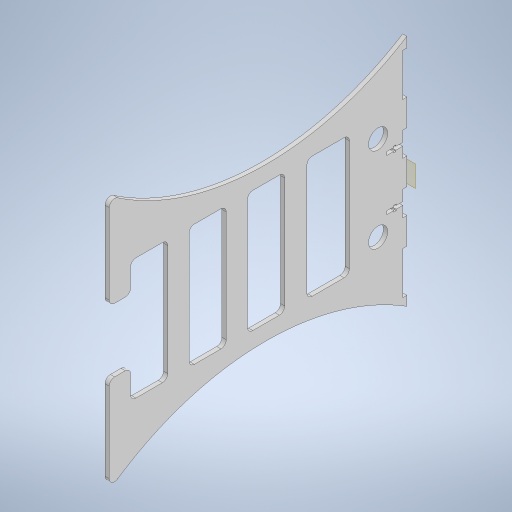
# Autodesk Inventor part: грань тела
Saved by Autodesk Inventor 2023.1 (Build 271208000, 208)
## iProperties
Created: 2024-11-21
Part Number: грань тела
Material: Типовые
Document SubType Name: Modeling
Designer: DELL
Density: 1 g/cm^3
Appearance: По умолчанию
Author: DELL
Autodesk Inventor part; units mm, degrees
ref_plane "YZ Plane" through (0, 0, 0) normal (1, 0, 0) x (0, 1, 0)
ref_plane "XZ Plane" through (0, 0, 0) normal (0, 1, 0) x (-1, 0, 0)
ref_plane "РабПлоскость1" through (0, 0, -4) normal (0, 0, 1) x (1, 0, 0)
sketch "Эскиз10" plane through (0, 0, 0) normal (1, 0, 0) x (0, 1, 0)
  line L0 (-120, -4) -> (120, -4) construction
  line L1 (120, -4) -> (120, 276) construction
  line L2 (110.389, 276) -> (-110.389, 276)
  line L3 (-120, 276) -> (-120, -4) construction
  line L4 (-110, -4) -> (110, -4)
  arc A0 (-110, -4) -> (-114.5368, 268.208) centre (-321.9309, 128.6096) ccw
  arc A1 (114.5368, 268.208) -> (110, -4) centre (321.9309, 128.6096) ccw
  arc A2 (114.5368, 268.208) -> (110.389, 276) centre (110.389, 271) ccw
  arc A3 (-110.389, 276) -> (-114.5368, 268.208) centre (-110.389, 271) ccw
  point P0 (0, 0)
  point P1 (0, -4)
  dimension "d50" = 240
  dimension "d51" = 280
  dimension "d52" = 220
  dimension "d53" = 250
  dimension "d54" = 250
  dimension "d55" = 5
  constraints: 10 end point, 10 point on circle, 4 centre point, 4 tangent, 2 horizontal, 2 midpoint, 2 parallel, 2 point on line, 1 equal radius, 1 perpendicular
  measures "d50" distance of L3.start L1.end
  measures "d51" distance of L1.end L0.end
  measures "d52" distance of L4.start L4.end
  measures "d53" radius of A0
  measures "d54" radius of A1
  measures "d55" radius of A2
extrude "Выдавливание6" add sketch "Эскиз10" along normal mid plane 4
sketch "Эскиз12" plane through (2, 0, 0) normal (1, 0, 0) x (0, 0, -1)
  line L0 (4.1067, -100.9593) -> (0, -100.9593)
  line L1 (0, -100.9593) -> (0, -60.9593)
  line L2 (0, -60.9593) -> (4, -60.9593)
  line L3 (4, 110) -> (4, -110) projected
  line L4 (4, -110) -> (4, 110) projected
  line L5 (4, -35.9593) -> (0, -35.9593)
  line L6 (0, -35.9593) -> (0, -12.5)
  line L7 (0, -12.5) -> (4, -12.5)
  line L8 (4, 12.5) -> (0, 12.5)
  line L9 (0, 12.5) -> (0, 35.5004)
  line L10 (0, 35.5004) -> (4, 35.5004)
  line L11 (4, 60.5004) -> (0, 60.5004)
  line L12 (0, 60.5004) -> (0, 100.5004)
  line L13 (0, 100.5004) -> (4, 100.5004)
  point P0 (0, 0)
  point P1 (4, 12.5)
  point P2 (4, 35.5004)
  point P3 (4, -35.9593)
  point P4 (4, -12.5)
  point P5 (4, -100.9593)
  constraints: 24 end point, 10 perpendicular, 7 point on line, 2 horizontal, 8 other
extrude "Выдавливание7" cut sketch "Эскиз12" against normal blind 4
sketch "Эскиз13" plane through (2, 0, 0) normal (1, 0, 0) x (0, 0, -1)
  line L0 (-15, -22.6546) -> (-15, -25.8046)
  line L1 (0, -25.7683) -> (0, -22.691)
  line L2 (0, -35.9593) -> (0, -12.5) projected
  line L3 (-6.1608, -27.016) -> (-8.4608, -27.016)
  line L4 (-8.4608, -21.516) -> (-6.1608, -21.516)
  line L5 (-15, -24.2296) -> (0, -24.2296) construction
  line L6 (0, -12.5) -> (0, -35.9593) projected
  line L7 (-8.4608, -27.016) -> (-8.4608, -25.8046)
  line L8 (-8.4608, -22.6546) -> (-8.4608, -21.516)
  line L9 (-15, -25.8046) -> (-8.4608, -25.8046)
  line L10 (-6.1608, -25.7683) -> (0, -25.7683)
  line L11 (-6.1608, -21.516) -> (-6.1608, -22.691)
  line L12 (-6.1608, -25.7683) -> (-6.1608, -27.016)
  line L13 (0, -22.691) -> (-6.1608, -22.691)
  line L14 (-8.4608, -22.6546) -> (-15, -22.6546)
  line L15 (0, 12.5) -> (0, 35.5004) projected
  line L16 (0, 18.7449) -> (0, 30.6124)
  line L17 (0, 22.4252) -> (0, 25.5752)
  line L18 (-15, 25.5752) -> (-15, 22.4252)
  line L19 (-8.65, 21.2502) -> (-6.35, 21.2502)
  line L20 (-6.35, 26.7502) -> (-8.65, 26.7502)
  line L21 (-15, 24.0002) -> (0, 24.0002) construction
  line L22 (-8.65, 26.7502) -> (-8.65, 25.5752)
  line L23 (-8.65, 22.4252) -> (-8.65, 21.2502)
  line L24 (-15, 22.4252) -> (-8.65, 22.4252)
  line L25 (-6.35, 22.4252) -> (0, 22.4252)
  line L26 (-6.35, 21.2502) -> (-6.35, 22.4252)
  line L27 (-6.35, 25.5752) -> (-6.35, 26.7502)
  line L28 (0, 25.5752) -> (-6.35, 25.5752)
  line L29 (-8.65, 25.5752) -> (-15, 25.5752)
  circle A0 centre (-23.1563, -40) radius 9
  line L30 (4, -35.9593) -> (4, -60.9593) projected
  line L31 (4, 35.5004) -> (4, 60.5004) projected
  line L32 (0, 0) -> (-64.5188, 0) construction
  circle A1 centre (-23.1563, 40) radius 9
  dimension "d60" = 15
  dimension "d61" = 3.15
  dimension "d62" = 2.3
  dimension "d63" = 5.5
  dimension "d64" = 6.35
  dimension "d70" = 15
  dimension "d71" = 3.15
  dimension "d72" = 2.3
  dimension "d73" = 5.5
  dimension "d77" = 18
  dimension "d114" = 80
  constraints: 56 end point, 20 parallel, 10 perpendicular, 8 midpoint, 7 horizontal, 2 centre point, 2 point on line, 1 symmetric about line, 1 other
  measures "d60" distance of L1.start L0.end
  measures "d61" distance of L0.end L0.start
  measures "d62" distance of L4.start L4.end
  measures "d63" distance of L3.end L4.start
  measures "d64" distance of point (0, -24.23) L11.end
  measures "d70" distance of L18.start L17.end
  measures "d71" distance of L17.end L17.start
  measures "d72" distance of L20.end L20.start
  measures "d73" distance of L20.start L19.end
  measures "d77" diameter of A0
  measures "d114" distance of A1.centre A0.centre
extrude "Выдавливание8" cut sketch "Эскиз13" against normal blind 4
sketch "Эскиз15" plane through (-2, 0, 0) normal (-1, 0, 0) x (0, 0, 1)
  line L0 (0, 75.3813) -> (0, -75.381) construction
  line L1 (0, 57.0002) -> (0, 61.0002) construction
  line L2 (0, 61.0002) -> (276, 61.0002) construction
  line L3 (276, 61.0002) -> (276, 57.0002) construction
  line L4 (276, 57.0002) -> (0, 57.0002) construction
  line L5 (0, -61.2296) -> (0, -57.2296) construction
  line L6 (0, -57.2296) -> (276, -57.2296) construction
  line L7 (276, -57.2296) -> (276, -61.2296) construction
  line L8 (276, -61.2296) -> (0, -61.2296) construction
  circle A0 centre (23.1563, 40) radius 9 construction
  circle A1 centre (23.1563, -40) radius 9 construction
  line L9 (50.1563, 57.0002) -> (50.1563, -52.2296) construction
  line L10 (116, 57.0002) -> (141, 57.0002)
  line L11 (146, 52.0002) -> (146, -52.2296)
  line L12 (141, -57.2296) -> (116, -57.2296)
  line L13 (111, -52.2296) -> (111, 52.0002)
  line L14 (226, 57.0002) -> (251, 57.0002)
  line L15 (251, -57.2296) -> (226, -57.2296)
  line L16 (221, -52.2296) -> (221, 52.0002)
  line L17 (276, 35.0002) -> (276, 110.389)
  line L18 (171, 57.0002) -> (196, 57.0002)
  line L19 (201, 52.0002) -> (201, -52.2296)
  line L20 (196, -57.2296) -> (171, -57.2296)
  line L21 (166, -52.2296) -> (166, 52.0002)
  line L22 (55.1563, 57.0002) -> (85.1563, 57.0002)
  line L23 (90.1563, 52.0002) -> (90.1563, -52.2296)
  line L24 (85.1563, -57.2296) -> (55.1563, -57.2296)
  line L25 (50.1563, -57.2296) -> (50.1563, 52.0002)
  arc A2 (55.1563, 57.0002) -> (50.1563, 52.0002) centre (55.1563, 52.0002) ccw
  arc A3 (90.1563, 52.0002) -> (85.1563, 57.0002) centre (85.1563, 52.0002) ccw
  arc A4 (50.1563, -52.2296) -> (55.1563, -57.2296) centre (55.1563, -52.2296) ccw
  arc A5 (85.1563, -57.2296) -> (90.1563, -52.2296) centre (85.1563, -52.2296) ccw
  arc A6 (116, 57.0002) -> (111, 52.0002) centre (116, 52.0002) ccw
  arc A7 (146, 52.0002) -> (141, 57.0002) centre (141, 52.0002) ccw
  arc A8 (111, -52.2296) -> (116, -57.2296) centre (116, -52.2296) ccw
  arc A9 (141, -57.2296) -> (146, -52.2296) centre (141, -52.2296) ccw
  arc A10 (171, 57.0002) -> (166, 52.0002) centre (171, 52.0002) ccw
  arc A11 (201, 52.0002) -> (196, 57.0002) centre (196, 52.0002) ccw
  arc A12 (196, -57.2296) -> (201, -52.2296) centre (196, -52.2296) ccw
  arc A13 (166, -52.2296) -> (171, -57.2296) centre (171, -52.2296) ccw
  arc A14 (226, 57.0002) -> (221, 52.0002) centre (226, 52.0002) ccw
  arc A15 (256, 52.0002) -> (251, 57.0002) centre (251, 52.0002) ccw
  arc A16 (251, -57.2296) -> (256, -52.2296) centre (251, -52.2296) ccw
  arc A17 (221, -52.2296) -> (226, -57.2296) centre (226, -52.2296) ccw
  line L26 (271, -29.9998) -> (261, -29.9998)
  line L27 (261, 30.0002) -> (271, 30.0002)
  line L28 (276, -13.2762) -> (255.9998, 30.0002) construction
  line L29 (255.9998, -29.9998) -> (276, 13.2766) construction
  line L30 (276, 41.3488) -> (276, 1056.4994)
  line L31 (276, 110.389) -> (276, -110.389) projected
  arc A18 (271, 30.0002) -> (276, 35.0002) centre (271, 35.0002) ccw
  line L32 (276, -34.9998) -> (276, -49)
  arc A19 (276, -34.9998) -> (271, -29.9998) centre (271, -34.9998) ccw
  line L33 (276, 57.0002) -> (276, -57.2296)
  line L34 (256, 52.0002) -> (256, 35.0002)
  line L35 (256, -34.9998) -> (256, -52.2296)
  arc A20 (256, 35.0002) -> (261, 30.0002) centre (261, 35.0002) ccw
  arc A21 (261, -29.9998) -> (256, -34.9998) centre (261, -34.9998) ccw
  point P0 (50.1563, -57.2296)
  point P1 (111, 57.0002)
  point P2 (146, -57.2296)
  point P3 (221, 57.0002)
  point P4 (256, -57.2296)
  point P5 (166, -0.1147)
  point P6 (166, 57.0002)
  point P7 (201, -57.2296)
  point P8 (90.1563, -57.2296)
  point P9 (50.1563, -52.2296)
  point P10 (269.8643, 0.0002)
  point P11 (276, 30.0002)
  point P12 (276, -29.9998)
  point P13 (256, 29.9998)
  point P14 (256, -29.9994)
  point P15 (276, -34.9998)
  point P16 (276, 35.0002)
  dimension "d99" = 27
  dimension "d101" = 35
  dimension "d107" = 35
  dimension "d108" = 20
  dimension "d109" = 20
  dimension "d110" = 40
  dimension "d111" = 5
  dimension "d117" = 5
  dimension "d118" = 5
  dimension "d119" = 5
  constraints: 68 end point, 41 tangent, 40 point on circle, 37 point on line, 20 centre point, 16 equal radius, 10 parallel, 6 perpendicular, 5 horizontal, 28 other
  measures "d99" distance from line of A0.centre L9
  measures "d101" distance between parallel lines of L11 L13
  measures "d107" distance between parallel lines of L21 L19
  measures "d108" distance between parallel lines of L16 L19
  measures "d109" distance between parallel lines of L21 L11
  measures "d110" distance from line of L25.start L23
  measures "d111" radius of A2
  measures "d117" radius of A18
  measures "d118" radius of A19
  measures "d119" radius of A20
extrude "Выдавливание10" cut sketch "Эскиз15" against normal blind 10
sketch "Эскиз17" plane through (-2, 0, 0) normal (-1, 0, 0) x (0, 0, 1)
  point P0 (0, 0)
